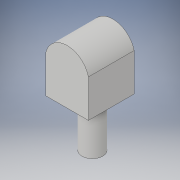
# Autodesk Inventor part: led
Saved by Autodesk Inventor 2019 (Build 230136000, 136)
## iProperties
Created: 2020-03-04
Part Number: led
Material: Generic
Document SubType Name: Modeling
Designer: ADMIN
Density: 1 g/cm^3
Appearance: Default
Author: ADMIN
Autodesk Inventor part; units mm, degrees
ref_plane "YZ Plane" through (0, 0, 0) normal (1, 0, 0) x (0, 1, 0)
ref_plane "XZ Plane" through (0, 0, 0) normal (0, 1, 0) x (-1, 0, 0)
ref_plane "XY Plane" through (0, 0, 0) normal (0, 0, 1) x (1, 0, 0)
sketch "Sketch1" plane through (0, 0, 0) normal (0, 0, 1) x (1, 0, 0)
  arc A0 (3.9123, 7.9106) -> (-5.3901, 7.9106) centre (-0.7389, 6.7419) ccw
  line L0 (3.9123, 7.9106) -> (-5.3901, 7.9106)
  line L1 (-5.3901, 7.9106) -> (3.9123, 7.9106)
  line L2 (3.9123, 7.9106) -> (3.9123, -0.326)
  line L3 (3.9123, -0.326) -> (-5.3901, -0.326)
  line L4 (-5.3901, -0.326) -> (-5.3901, 7.9106)
  point P0 (0, 0)
  constraints: 10 end point, 2 horizontal, 2 parallel, 2 point on circle, 1 centre point, 1 perpendicular
extrude "Extrusion1" add sketch "Sketch1" along normal blind 10
sketch "Sketch2" plane through (-5.3901, -0.326, 0) normal (0, -1, 0) x (1, 0, 0)
  circle A0 centre (5.3901, 5.2158) radius 2.2686
  point P0 (5.3901, 0)
  constraints: 1 centre point
extrude "Extrusion2" add sketch "Sketch2" along normal blind 10
body "Solid1"
